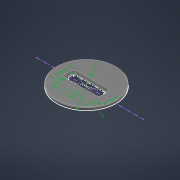
# Autodesk Inventor part: фланец2
Saved by Autodesk Inventor 2022 (Build 260153070, 153G)
## iProperties
Created: 2022-02-03
Part Number: фланец2
Material: Термопластическая смола
Document SubType Name: Modeling
Designer: kalugin_a
Density: 1.28 g/cm^3
Appearance: Гладкая — черная
Author: kalugin_a
Autodesk Inventor part; units mm, degrees
ref_plane "YZ Plane" through (0, 0, 0) normal (1, 0, 0) x (0, 1, 0)
ref_plane "XZ Plane" through (0, 0, 0) normal (0, 1, 0) x (-1, 0, 0)
sketch "Эскиз1" plane through (0, 0, 0) normal (0, 1, 0) x (-1, 0, 0)
  circle A0 centre (0, 0) radius 52.5
  line L0 (89.6506, 0) -> (-102.8587, 0)
  line L1 (-27, -7.5) -> (27, -7.5)
  line L2 (30, -4.5) -> (30, 4.5)
  line L3 (27, 7.5) -> (-27, 7.5)
  line L4 (-30, 4.5) -> (-30, -4.5)
  line L5 (-30, -7.5) -> (30, 7.5) construction
  line L6 (30, -7.5) -> (-30, 7.5) construction
  arc A1 (30, 4.5) -> (27, 7.5) centre (27, 4.5) ccw
  arc A2 (27, -7.5) -> (30, -4.5) centre (27, -4.5) ccw
  arc A3 (-27, 7.5) -> (-30, 4.5) centre (-27, 4.5) ccw
  arc A4 (-30, -4.5) -> (-27, -7.5) centre (-27, -4.5) ccw
  line L7 (33, -12) -> (-33, -12)
  line L8 (-35, -10) -> (-35, 10)
  line L9 (-33, 12) -> (33, 12)
  line L10 (35, 10) -> (35, -10)
  line L11 (35, -12) -> (-32.3514, 11.0919) construction
  line L12 (-35, -12) -> (35, 12) construction
  arc A5 (-33, 12) -> (-35, 10) centre (-33, 10) ccw
  arc A6 (-35, -10) -> (-33, -12) centre (-33, -10) ccw
  arc A7 (33, -12) -> (35, -10) centre (33, -10) ccw
  arc A8 (35, 10) -> (33, 12) centre (33, 10) ccw
  point P0 (-35, 12)
  dimension "d0" = 105
  dimension "d1" = 60
  dimension "d2" = 15
  dimension "d3" = 3
  dimension "d4" = 3
  dimension "d13" = 70
  dimension "d14" = 24
  dimension "d15" = 2
  constraints: 27 end point, 18 point on line, 16 point on circle, 16 tangent, 9 centre point, 4 equal radius, 4 parallel, 3 horizontal, 3 midpoint, 2 perpendicular, 1 coincident
  measures "d0" diameter of A0
  measures "d1" distance of L6.end L5.end
  measures "d2" distance of L5.end L6.start
  measures "d3" radius of A1
  measures "d4" radius of A2
  measures "d13" distance of point (-35, 12) L12.end
  measures "d14" distance of L12.start point (-35, 12)
  measures "d15" radius of A5
extrude "Выдавливание1" add sketch "Эскиз1" along normal blind 5 contours L0 L10 A8 L9 A5 L8 A0 | A0 L0 L8 A6 L7 A7 L10 | L10 A7 L7 A6 L8 L0 L4 A4 L1 A2 L2 | L0 L2 A1 L3 A3 L4 L8 A5 L9 A8 L10
chamfer "Фаска1" distance 3 angle 45 8 edges at (0, 5, 7.5) (-29.1213, 5, 6.6213) (-30, 5, 0) (-29.1213, 5, -6.6213) (0, 5, -7.5) (29.1213, 5, -6.6213) (30, 5, 0) (29.1213, 5, 6.6213)
chamfer "Фаска2" distance 1 angle 45 1 edges at (52.5, 5, 0)
extrude "Выдавливание2" cut sketch "Эскиз1" along normal blind 1.5 contours L10 A7 L7 A6 L8 L0 L4 A4 L1 A2 L2 | L0 L2 A1 L3 A3 L4 L8 A5 L9 A8 L10 | L2 A2 L1 A4 L4 L0 | L0 L4 A3 L3 A1 L2
ref_plane "РабПлоскость1" through (0, 2.5, 0) normal (0, -1, 0) x (1, 0, 0)
